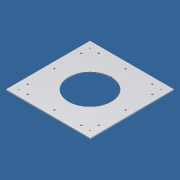
# Autodesk Inventor part: J002446_1
Saved by Autodesk Inventor 2015 SP1 (Build 190203100, 203)
## iProperties
Created: 2012-08-06
Material: UHMW, WHITE
Vendor: HHMI: JFRC - ID&F
Document SubType Name: Modeling
Designer: NEGRASHOVI
Density: 0.93 g/cm^3
Mass: 97.1286 g
Surface Area: 783.642 cm^2
Volume: 104.439 cm^3
Description: CHAMBER SPACER SHALLOW
Appearance: Smooth - White
Part Number: J002446_1
Project: P-270901
RuleStatus: InUse
AfterDocSave0: file://Part Number Cleaner
LAB/DEPT: COMMON
REQUESTING SCIENTIST: COMMON
SURFACE ROUGHNESS: 32 ra
DESIGN DEPARTMENT: HHMI: JRC - ID&F
SPECIAL FINISH: NONE
ALTERED ITEM PART NUMBER: N/A
ALTERED ITEM VENDOR: N/A
ALTERED ITEM DESCRIPTION: N/A
Author: NEGRASHOVI
Revision Number: A
Autodesk Inventor part; units mm, degrees
ref_plane "YZ Plane" through (0, 0, 0) normal (1, 0, 0) x (0, 1, 0)
ref_plane "XZ Plane" through (0, 0, 0) normal (0, 1, 0) x (-1, 0, 0)
ref_plane "XY Plane" through (0, 0, 0) normal (0, 0, 1) x (1, 0, 0)
sketch "Sketch1" plane through (0, 0, 0) normal (0, 0, 1) x (1, 0, 0)
  line L0 (-107.95, 107.95) -> (107.95, 107.95)
  line L1 (107.95, 107.95) -> (107.95, -107.95)
  line L2 (107.95, -107.95) -> (-107.95, -107.95)
  line L3 (-107.95, -107.95) -> (-107.95, 107.95)
  line L4 (-107.95, -107.95) -> (107.95, 107.95) construction
  point P0 (0, 0)
  point P1 (0, 0)
  dimension "d0" = 215.9
  dimension "d1" = 215.9
  constraints: 10 end point, 2 parallel, 1 coincident, 1 horizontal, 1 midpoint, 1 perpendicular
  measures "d0" distance of L0.start L0.end
  measures "d1" distance of L2.end L0.start
extrude "Extrusion1" add sketch "Sketch1" along normal blind 3
sketch "Sketch3" plane through (0, 0, 0) normal (0, 0, -1) x (-1, 0, 0)
  line L0 (256.032, 0) -> (-256.032, 0) construction
  line L1 (0, -256.032) -> (0, 256.032) construction
  line L2 (-101.6, 101.6) -> (101.6, 101.6) construction
  line L3 (-101.6, -101.6) -> (101.6, -101.6) construction
  line L4 (101.6, 101.6) -> (-101.6, -101.6) construction
  line L5 (101.6, -101.6) -> (-101.6, 101.6) construction
  arc A0 (-90.3175, 92.5625) -> (-92.5625, 92.5625) centre (-91.44, 91.44) ccw
  arc A1 (-90.3175, 92.5625) -> (0, 55.1518) centre (0, 182.88) ccw
  line L6 (-91.44, 91.44) -> (0, 182.88) construction
  arc A2 (-92.5625, 92.5625) -> (-92.5625, 90.3175) centre (-91.44, 91.44) ccw
  arc A3 (-55.1518, 0) -> (-92.5625, 90.3175) centre (-182.88, 0) ccw
  arc A4 (92.5625, 92.5625) -> (90.3175, 92.5625) centre (91.44, 91.44) ccw
  arc A5 (0, 55.1518) -> (90.3175, 92.5625) centre (0, 182.88) ccw
  arc A6 (92.5625, 90.3175) -> (55.1518, 0) centre (182.88, 0) ccw
  arc A7 (92.5625, 90.3175) -> (92.5625, 92.5625) centre (91.44, 91.44) ccw
  arc A8 (-92.5625, -92.5625) -> (-90.3175, -92.5625) centre (-91.44, -91.44) ccw
  arc A9 (0, -55.1518) -> (-90.3175, -92.5625) centre (0, -182.88) ccw
  arc A10 (-92.5625, -90.3175) -> (-55.1518, 0) centre (-182.88, 0) ccw
  arc A11 (-92.5625, -90.3175) -> (-92.5625, -92.5625) centre (-91.44, -91.44) ccw
  arc A12 (55.1518, 0) -> (92.5625, -90.3175) centre (182.88, 0) ccw
  arc A13 (90.3175, -92.5625) -> (0, -55.1518) centre (0, -182.88) ccw
  arc A14 (90.3175, -92.5625) -> (92.5625, -92.5625) centre (91.44, -91.44) ccw
  arc A15 (92.5625, -92.5625) -> (92.5625, -90.3175) centre (91.44, -91.44) ccw
  point P0 (0, 0)
  dimension "d168" = 3.175
  dimension "d169" = 91.44
  constraints: 32 point on circle, 19 symmetric about line, 16 centre point, 14 end point, 5 point on line, 2 perpendicular, 1 tangent, 14 other
  measures "d168" diameter of A0
  measures "d169" horizontal distance of L6.start point (0, 0)
extrude "Extrusion5" cut sketch "Sketch3" against normal blind 0.7
sketch "Sketch6" plane through (0, 0, 0.7) normal (0, 0, -1) x (-1, 0, 0)
  circle A0 centre (0, 0) radius 55.1518
  arc A1 (-90.3175, 92.5625) -> (-92.5625, 90.3175) centre (-91.44, 91.44) ccw
  arc A2 (-92.5625, -90.3175) -> (-92.5625, 90.3175) centre (-182.88, 0) ccw
  arc A3 (-92.5625, -90.3175) -> (-90.3175, -92.5625) centre (-91.44, -91.44) ccw
  arc A4 (90.3175, -92.5625) -> (-90.3175, -92.5625) centre (0, -182.88) ccw
  arc A5 (90.3175, -92.5625) -> (92.5625, -90.3175) centre (91.44, -91.44) ccw
  arc A6 (92.5625, 90.3175) -> (92.5625, -90.3175) centre (182.88, 0) ccw
  arc A7 (92.5625, 90.3175) -> (90.3175, 92.5625) centre (91.44, 91.44) ccw
  arc A8 (-90.3175, 92.5625) -> (90.3175, 92.5625) centre (0, 182.88) ccw
  arc A9 (-90.3175, 92.5625) -> (90.3175, 92.5625) centre (0, 182.88) ccw
  point P0 (0, 0)
  constraints: 18 point on circle, 10 centre point, 1 coincident, 1 tangent
extrude "Extrusion6" cut sketch "Sketch6" against normal up to next contours A0
sketch "Sketch11" plane through (0, 0, 3) normal (0, 0, 1) x (1, 0, 0)
  line L0 (-91.44, 91.44) -> (91.44, 91.44) construction
  line L1 (91.44, 91.44) -> (91.44, -91.44) construction
  line L2 (91.44, -91.44) -> (-91.44, -91.44) construction
  line L3 (-91.44, -91.44) -> (-91.44, 91.44) construction
  line L4 (-151.13, 0) -> (151.13, 0) construction
  line L5 (0, -151.13) -> (0, 151.13) construction
  point P0 (0, 0)
  dimension "d170" = 182.88
  dimension "d171" = 182.88
  constraints: 8 end point, 4 coincident, 2 parallel, 1 horizontal, 1 perpendicular, 2 other
  measures "d170" distance of L0.start L0.end
  measures "d171" distance between parallel lines of L2 L0
hole "Hole15" at (-91.44, 91.44, 3) at (91.44, 91.44, 3) at (91.44, -91.44, 3) at (-91.44, -91.44, 3) direction (0, 0, -1) diameter 3.175 end through all
sketch "Sketch13" plane through (0, 0, 3) normal (0, 0, 1) x (1, 0, 0)
  line L0 (-91.44, -91.44) -> (91.44, -91.44) construction
  line L1 (91.44, -91.44) -> (91.44, 91.44) construction
  line L2 (91.44, 91.44) -> (-91.44, 91.44) construction
  line L3 (-91.44, 91.44) -> (-91.44, -91.44) construction
  line L4 (-91.44, -91.44) -> (91.44, 91.44) construction
  line L5 (-151.13, 0) -> (151.13, 0) construction
  line L6 (0, -151.13) -> (0, 151.13) construction
  point P0 (0, 0)
  point P1 (0, 0)
  point P2 (-68.58, 91.44)
  point P3 (0, 91.44)
  point P4 (68.58, 91.44)
  point P5 (91.44, 68.58)
  point P6 (91.44, 0)
  point P7 (91.44, -68.58)
  point P8 (68.58, -91.44)
  point P9 (0, -91.44)
  point P10 (-68.58, -91.44)
  point P11 (-91.44, -68.58)
  point P12 (-91.44, 0)
  point P13 (-91.44, 68.58)
  dimension "d302" = 182.88
  dimension "d303" = 182.88
  dimension "d304" = 22.86
  dimension "d305" = 22.86
  constraints: 12 point on line, 10 end point, 6 symmetric about line, 5 midpoint, 2 parallel, 1 coincident, 1 horizontal, 1 perpendicular
  measures "d302" distance of L1.end L2.end
  measures "d303" distance of L0.end L1.end
  measures "d304" distance from line of point (-68.58, 91.44) L3
  measures "d305" distance from line of point (-91.44, 68.58) L2
hole "Hole29" at (-68.58, 91.44, 3) at (0, 91.44, 3) at (68.58, 91.44, 3) at (91.44, 68.58, 3) at (91.44, 0, 3) at (91.44, -68.58, 3) at (68.58, -91.44, 3) at (0, -91.44, 3) at (-68.58, -91.44, 3) at (-91.44, -68.58, 3) at (-91.44, 0, 3) at (-91.44, 68.58, 3) direction (0, 0, -1) diameter 4.4958 end through all clearance for "Flat Head Machine Screw (82)" size "#8" standard "Ansi Unified Screw Threads"
sketch "Sketch14" plane through (0, 0, 3) normal (0, 0, 1) x (1, 0, 0)
  circle A0 centre (0, 0) radius 55.1518 projected
  line L0 (0, -151.13) -> (0, 151.13) construction
  circle A1 centre (0, 55.1518) radius 1.5875
  point P0 (0, 0)
  dimension "d313" = 3.175
  constraints: 1 centre point, 1 point on line, 1 vertical alignment, 1 other
  measures "d313" diameter of A1
extrude "Extrusion9" cut sketch "Sketch14" against normal through all contours A1 A0 | A0 A1 picked at (0.0632, 54.6247) picked at (0.0603, 55.6758)
equation "\"d1\" = d0"
body "Solid1"
